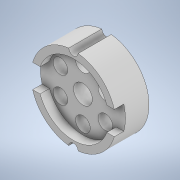
# Autodesk Inventor part: light_hole
Saved by Autodesk Inventor 2022 (Build 260153000, 153)
## iProperties
Created: 2021-07-10
Part Number: light_hole
Material: 常规
Document SubType Name: Modeling
Designer: Ricardo
Density: 1 g/cm^3
Appearance: 默认
Author: Ricardo
Autodesk Inventor part; units mm, degrees
ref_plane "YZ Plane" through (0, 0, 0) normal (1, 0, 0) x (0, 1, 0)
ref_plane "XZ Plane" through (0, 0, 0) normal (0, 1, 0) x (-1, 0, 0)
ref_plane "XY Plane" through (0, 0, 0) normal (0, 0, 1) x (1, 0, 0)
sketch "草图3" plane through (0, 0, 0) normal (0, 0, 1) x (1, 0, 0)
  circle A0 centre (0, 0) radius 2
  circle A1 centre (0, 0) radius 7.5
  circle A2 centre (0, 0) radius 5.5
  circle A3 centre (0, 5.5) radius 1.55
  circle A4 centre (-4.7631, 2.75) radius 1.55
  circle A5 centre (-4.7631, -2.75) radius 1.55
  circle A6 centre (0, -5.5) radius 1.55
  circle A7 centre (4.7631, -2.75) radius 1.55
  circle A8 centre (4.7631, 2.75) radius 1.55
  arc A9 (0.9985, -8.9444) -> (-0.9985, -8.9444) centre (0, -9) ccw
  arc A10 (-0.9985, 8.9444) -> (-8.6458, 2.5) centre (0, 0) ccw
  arc A11 (0.9985, -8.9444) -> (0.9985, 8.9444) centre (0, 0) ccw
  arc A12 (-0.9985, 8.9444) -> (0.9985, 8.9444) centre (0, 9) ccw
  arc A13 (-8.9128, 1.25) -> (-8.9303, 1.1176) centre (0, 0) ccw
  arc A14 (-8.9128, -1.25) -> (-0.9985, -8.9444) centre (0, 0) ccw
  line L0 (-6.7281, -2.5) -> (-9.7719, 2.5) construction
  line L1 (-9.7719, -2.5) -> (-6.7281, 2.5) construction
  line L2 (6.8134, -2.5) -> (9.6866, 2.5) construction
  line L3 (9.6866, -2.5) -> (6.8134, 2.5) construction
  arc A15 (-8.6458, 2.5) -> (-8.9128, 1.25) centre (0, 0) ccw
  arc A16 (-8.9303, 1.1176) -> (-8.9128, -1.25) centre (0, 0) ccw
  line L4 (-8.6458, 2.5) -> (-7.0711, 2.5)
  line L5 (-7.0711, -2.5) -> (-8.6458, -2.5)
  line L6 (7.0711, -2.5) -> (8.6458, -2.5)
  line L7 (8.6458, 2.5) -> (7.0711, 2.5)
  point P0 (-8.25, 0)
  point P1 (8.25, 0)
  dimension "d30" = 11
  dimension "d28" = 4
  dimension "d29" = 15
  dimension "d31" = 3.1
  dimension "d34" = 360
  dimension "d38" = 2
  dimension "d43" = 5
  dimension "d44" = 5
  constraints: 25 point on circle, 16 centre point, 16 end point, 4 coincident, 4 midpoint, 2 horizontal, 2 parallel, 1 point on line, 1 vertical alignment, 15 other
  measures "d28" diameter of A0
  measures "d29" diameter of A1
  measures "d31" diameter of A3
  measures "d38" diameter of A9
  measures "d43" distance of L1.start L0.end
  measures "d44" distance of L2.end L3.start
extrude "拉伸4" add sketch "草图3" along normal blind 5 contours A1 | A2 A7 A6 A5 A4 A3 A8
extrude "拉伸5" add sketch "草图3" along normal blind 7 contours A1 L4 A10 A12 A11 L7 | L6 A11 A9 A14 L5 A1
extrude "拉伸6" add sketch "草图3" along normal blind 5 contours A1 L7 A11 L6 | A1 L5 A14 A16 A13 A15 L4
